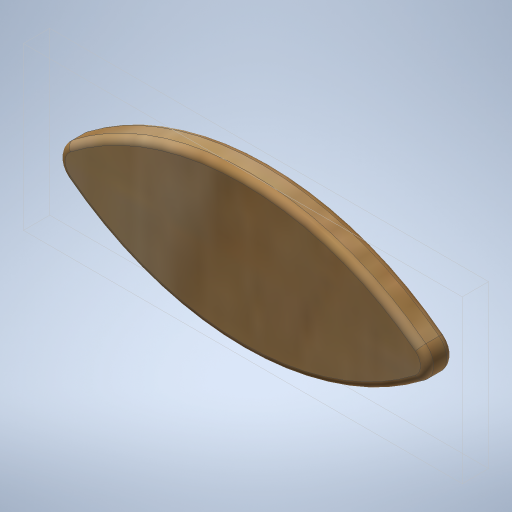
# Autodesk Inventor part: Lamello Biscuit 20
Saved by Autodesk Inventor 2024 (Build 280153000, 153)
## iProperties
Created: 2016-02-26
Part Number: Lamello Biscuit 20
Material: SW01
Description: Lamello Bisquit
Document SubType Name: Modeling
Designer: SauliusD
Density: 0.721 g/cm^3
Appearance: SW01
Author: SauliusD
Autodesk Inventor part; units mm, degrees
ref_plane "YZ Plane" through (0, 0, 0) normal (1, 0, 0) x (0, 1, 0)
ref_plane "XZ Plane" through (0, 0, 0) normal (0, 1, 0) x (-1, 0, 0)
ref_plane "XY Plane" through (0, 0, 0) normal (0, 0, 1) x (1, 0, 0)
sketch "Sketch1" plane through (0, 0, 0) normal (0, 0, 1) x (1, 0, 0)
  line L0 (-62.3, 0) -> (62.3, 0) construction
  line L1 (33.35, 2) -> (-33.35, 2)
  line L2 (-33.35, 2) -> (-33.35, -2)
  line L3 (-33.35, -2) -> (33.35, -2)
  line L4 (33.35, -2) -> (33.35, 2)
  point P0 (0, 0)
  point P1 (0, 2)
  point P2 (33.35, 0)
  dimension "d0" = 4
  dimension "d1" = 66.7
  constraints: 8 end point, 2 midpoint, 2 parallel, 1 horizontal, 1 perpendicular, 1 point on line, 1 vertical alignment
  measures "d0" distance of L1.end L2.end
  measures "d1" distance of L2.end L3.end
extrude "Groove Extrusion1" add sketch "Sketch1" along normal mid plane 24.6
sketch "Sketch2" plane through (0, 0, 0) normal (0, 1, 0) x (-1, 0, 0)
  line L0 (28, -11.5) -> (-28, -11.5) construction
  line L1 (-28, -11.5) -> (-28, 11.5) construction
  line L2 (-28, 11.5) -> (28, 11.5) construction
  line L3 (28, 11.5) -> (28, -11.5) construction
  line L4 (28, -11.5) -> (-28, 11.5) construction
  line L5 (-28, -11.5) -> (28, 11.5) construction
  arc A0 (26.8286, 2.3783) -> (-26.8286, 2.3783) centre (0, -32.5147) ccw
  arc A1 (-26.8286, -2.3783) -> (26.8286, -2.3783) centre (0, 32.5147) ccw
  arc A2 (26.8286, -2.3783) -> (26.8286, 2.3783) centre (25, 0) ccw
  arc A3 (-26.8286, 2.3783) -> (-26.8286, -2.3783) centre (-25, 0) ccw
  point P0 (0, 0)
  point P1 (0, 0)
  point P2 (0, 0)
  dimension "d7" = 3
  dimension "d8" = 56
  dimension "d9" = 23
  constraints: 12 end point, 8 point on circle, 8 tangent, 4 centre point, 4 midpoint, 2 parallel, 2 vertical alignment, 1 equal radius, 1 horizontal, 1 perpendicular
  measures "d7" radius of A3
  measures "d8" distance of L1.end L2.end
  measures "d9" distance of L2.end L0.start
extrude "Lamello Extrusion3" add sketch "Sketch2" along normal up to surface (4 mm away) from surface at -2 separate body
fillet "Lamello Fillet1" radius 1 8 edges at (28, -2, 0) (0, -2, -11.5) (-28, -2, 0) (0, -2, 11.5) (-28, 2, 0) (0, 2, -11.5) (28, 2, 0) (0, 2, 11.5)
equation "\"d0\" = Groove_T"
equation "\"d1\" = Groove_L"
equation "\"d3\" = 2 * Groove_W"
equation "\"d8\" = Lamello_L"
equation "\"d9\" = Lamello_W"
equation "\"d10\" = 2 * Groove_W"
equation "\"Groove_W\" = 12.3"
equation "\"Groove_T\" = 4"
equation "\"Groove_L\" = 66.7"
equation "\"Lamello_W\" = 23"
equation "\"Lamello_L\" = 56"
equation "\"Lamello_T\" = 4"
